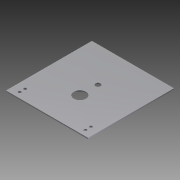
# Autodesk Inventor part: SensorPlatta
Saved by Autodesk Inventor 2014 (Build 180170000, 170)
## iProperties
Created: 2014-02-18
Part Number: SensorPlatta
Material: Generic
Document SubType Name: Sheet Metal
Designer: Pinkponk
Density: 1 g/cm^3
Sheet Metal Rule: Default_mm
Appearance: Default
Author: Pinkponk
Autodesk Inventor part; units mm, degrees
ref_plane "YZ Plane" through (0, 0, 0) normal (1, 0, 0) x (0, 1, 0)
ref_plane "XZ Plane" through (0, 0, 0) normal (0, 1, 0) x (-1, 0, 0)
ref_plane "XY Plane" through (0, 0, 0) normal (0, 0, 1) x (1, 0, 0)
sketch "Sketch1" plane through (0, 0, 0) normal (0, 0, 1) x (1, 0, 0)
  line L0 (0, 0) -> (150, 0)
  line L1 (150, 0) -> (150, 157)
  line L2 (150, 157) -> (0, 157)
  line L3 (0, 157) -> (0, 0)
  dimension "d0" = 157
  dimension "d1" = 150
  measures "d0" distance between parallel lines of L0 L2
  measures "d1" distance of L1.end L2.end
extrude "Plate1" add sketch "Sketch1" along normal blind 2
sketch "Sketch2" plane through (0, 0, 2) normal (0, 0, 1) x (1, 0, 0)
  line L0 (0, 0) -> (0, 157) projected
  line L1 (0, 157) -> (150, 157) projected
  circle A0 centre (75, 60) radius 11
  line L2 (150, 0) -> (0, 0) projected
  line L3 (150, 157) -> (150, 0) projected
  circle A1 centre (15, 10) radius 2.5
  circle A2 centre (15, 20) radius 2.5
  line L4 (75, 0) -> (75, 157) construction
  circle A3 centre (135, 10) radius 2.5
  circle A4 centre (135, 20) radius 2.5
  circle A5 centre (75, 93) radius 4.5
  point P0 (0, 78.5)
  dimension "d3" = 22
  dimension "d6" = 5
  dimension "d7" = 5
  dimension "d8" = 15
  dimension "d9" = 10
  dimension "d10" = 10
  dimension "d11" = 9
  dimension "d12" = 33
  dimension "d13" = 60
  constraints: 6 centre point, 3 midpoint, 2 end point, 2 symmetric about line, 2 vertical alignment, 1 parallel, 1 point on line, 2 other
  measures "d3" diameter of A0
  measures "d6" diameter of A2
  measures "d7" diameter of A1
  measures "d8" distance from line of L0 A1.centre
  measures "d9" distance from line of L2 A1.centre
  measures "d10" distance of A2.centre A1.centre
  measures "d11" diameter of A5
  measures "d12" distance of A0.centre A5.centre
  measures "d13" distance from line of L2 A0.centre
extrude "Extrusion1" cut sketch "Sketch2" against normal through all contours A0 | A1 | A2 | A3 | A4 | A5
equation "\"BendRadius\" = Thickness"
equation "\"BendReliefWidth\" = Thickness"
equation "\"BendReliefDepth\" = 0.5 * Thickness"
equation "\"CornerReliefSize\" = 4 * Thickness"
equation "\"MinimumRemnant\" = 2 * Thickness"
equation "\"TransitionRadius\" = BendRadius"
equation "\"JacobiRadiusSize\" = BendRadius"
equation "\"GapSize\" = Thickness"
equation "\"d2\" = BendRadius"
equation "\"Thickness\" = 2"
body "Solid1"
